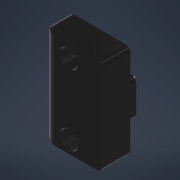
# Autodesk Inventor part: USBCClamp
Saved by Autodesk Inventor 2022 (Build 260153000, 153)
## iProperties
Created: 2021-10-03
Part Number: USBCClamp
Material: Generic
Document SubType Name: Modeling
Designer: trl121
Density: 1 g/cm^3
Appearance: Default
Author: trl121
Autodesk Inventor part; units mm, degrees
ref_plane "YZ Plane" through (0, 0, 0) normal (1, 0, 0) x (0, 1, 0)
ref_plane "XZ Plane" through (0, 0, 0) normal (0, 1, 0) x (-1, 0, 0)
ref_plane "Work Plane1" through (-169.39, -1.905, -0.5195) normal (-1, 0, 0) x (0, -1, 0)
sketch "Sketch1" plane through (-169.39, -1.905, -0.5195) normal (-1, 0, 0) x (0, -1, 0)
  arc A0 (80.1963, 0.7214) -> (80.1963, 3.3714) centre (80.1963, 2.0464) ccw construction
  line L0 (80.1963, 0.7214) -> (74.5063, 0.7214) construction
  arc A1 (74.5063, 3.3714) -> (74.5063, 0.7214) centre (74.5063, 2.0464) ccw construction
  line L1 (74.5063, 3.3714) -> (80.1963, 3.3714) construction
  line L2 (83.7013, -1.7636) -> (71.0013, -1.7636) construction
  arc A2 (83.7013, -1.7636) -> (84.9713, -0.4936) centre (83.7013, -0.4936) ccw construction
  line L3 (84.9713, 5.8564) -> (84.9713, -0.4936) construction
  line L4 (69.7313, -0.4936) -> (69.7313, 5.8564) construction
  arc A3 (69.7313, -0.4936) -> (71.0013, -1.7636) centre (71.0013, -0.4936) ccw construction
  line L5 (69.7313, 5.8564) -> (60.8413, 5.8564) construction
  line L6 (60.8413, 5.8564) -> (60.8413, 12.4375) construction
  line L7 (60.8413, 17.5175) -> (60.8413, 12.4375) construction
  line L8 (93.8613, 5.8564) -> (84.9713, 5.8564) construction
  line L9 (93.8613, 12.4375) -> (93.8613, 5.8564) construction
  line L10 (93.8613, 12.4375) -> (93.8613, 17.5175) construction
  line L11 (93.6613, 17.5175) -> (93.6613, 7.8564)
  line L12 (93.6613, 7.8564) -> (83.7013, 7.8564)
  line L13 (61.0413, 17.5175) -> (61.0413, 7.8564)
  line L14 (61.0413, 7.8564) -> (71.0013, 7.8564)
  line L15 (61.0413, 17.5175) -> (93.6613, 17.5175)
  line L16 (80.1963, 2.0464) -> (74.5063, 2.0464) construction
  line L17 (83.7013, 5.8564) -> (71.0013, 5.8564)
  line L18 (83.7013, 7.8564) -> (83.7013, 5.8564)
  line L19 (71.0013, 5.8564) -> (71.0013, 7.8564)
  point P0 (-1.905, 0.5195)
  dimension "d0" = 2
  dimension "d1" = 0.2
  dimension "d2" = 0.2
  dimension "d3" = 1.27
  dimension "d4" = 1.27
  constraints: 18 end point, 3 perpendicular, 3 vertical, 2 horizontal, 2 horizontal alignment, 2 vertical alignment, 1 collinear, 1 parallel, 1 other
  measures "d0" distance between parallel lines of L8 L12
  measures "d1" distance between parallel lines of L9 L11
  measures "d2" distance between parallel lines of L6 L13
  measures "d3" distance between parallel lines of L18 L3
  measures "d4" distance between parallel lines of L19 L4
extrude "Body" add sketch "Sketch1" against normal blind 20.955
sketch "Sketch2" plane through (-169.39, -95.5663, 16.998) normal (0, 0, 1) x (1, 0, 0)
  circle A0 centre (9.525, 4.245) radius 1.6 projected
  circle A1 centre (9.525, 28.375) radius 1.6 projected
  point P0 (169.39, 95.5663)
extrude "ScrewHoles" cut sketch "Sketch2" against normal through all
sketch "Sketch3" plane through (-169.39, -95.5663, 16.998) normal (0, 0, 1) x (1, 0, 0)
  circle A0 centre (9.525, 4.245) radius 1.6 construction
  circle A1 centre (9.525, 4.245) radius 3.175
  circle A2 centre (9.525, 28.375) radius 3.175
  circle A3 centre (9.525, 28.375) radius 1.6 construction
  point P0 (169.39, 95.5663)
  dimension "d9" = 6.35
  constraints: 2 centre point, 1 coincident, 1 concentric, 1 equal radius
  measures "d9" diameter of A1
extrude "ScrewHeadCut" cut sketch "Sketch3" against normal blind 4.445
sketch "Sketch4" plane through (-169.39, -85.6063, 5.3369) normal (0, 0, -1) x (-1, 0, 0)
  line L0 (0, 12.7) -> (0, 0) construction
  line L1 (0, 12.7) -> (-20.955, 12.7) construction
  line L2 (-20.955, 0) -> (-20.955, 12.7) construction
  line L3 (0, 0) -> (-20.955, 0) construction
  line L4 (-0.6985, 12.319) -> (-1.9685, 12.319)
  line L5 (-1.9685, 12.319) -> (-1.9685, 11.049)
  line L6 (-1.9685, 11.049) -> (-0.6985, 11.049)
  line L7 (-0.6985, 11.049) -> (-0.6985, 12.319)
  line L8 (-2.2225, 12.319) -> (-3.4925, 12.319)
  line L9 (-3.4925, 12.319) -> (-3.4925, 11.049)
  line L10 (-3.4925, 11.049) -> (-2.2225, 11.049)
  line L11 (-2.2225, 11.049) -> (-2.2225, 12.319)
  line L12 (-3.7465, 12.319) -> (-5.0165, 12.319)
  line L13 (-5.0165, 12.319) -> (-5.0165, 11.049)
  line L14 (-5.0165, 11.049) -> (-3.7465, 11.049)
  line L15 (-3.7465, 11.049) -> (-3.7465, 12.319)
  line L16 (-5.2705, 12.319) -> (-6.5405, 12.319)
  line L17 (-6.5405, 12.319) -> (-6.5405, 11.049)
  line L18 (-6.5405, 11.049) -> (-5.2705, 11.049)
  line L19 (-5.2705, 11.049) -> (-5.2705, 12.319)
  line L20 (-6.7945, 12.319) -> (-8.0645, 12.319)
  line L21 (-8.0645, 12.319) -> (-8.0645, 11.049)
  line L22 (-8.0645, 11.049) -> (-6.7945, 11.049)
  line L23 (-6.7945, 11.049) -> (-6.7945, 12.319)
  line L24 (-8.3185, 12.319) -> (-9.5885, 12.319)
  line L25 (-9.5885, 12.319) -> (-9.5885, 11.049)
  line L26 (-9.5885, 11.049) -> (-8.3185, 11.049)
  line L27 (-8.3185, 11.049) -> (-8.3185, 12.319)
  line L28 (-9.8425, 12.319) -> (-11.1125, 12.319)
  line L29 (-11.1125, 12.319) -> (-11.1125, 11.049)
  line L30 (-11.1125, 11.049) -> (-9.8425, 11.049)
  line L31 (-9.8425, 11.049) -> (-9.8425, 12.319)
  line L32 (-11.3665, 12.319) -> (-12.6365, 12.319)
  line L33 (-12.6365, 12.319) -> (-12.6365, 11.049)
  line L34 (-12.6365, 11.049) -> (-11.3665, 11.049)
  line L35 (-11.3665, 11.049) -> (-11.3665, 12.319)
  line L36 (-12.8905, 12.319) -> (-14.1605, 12.319)
  line L37 (-14.1605, 12.319) -> (-14.1605, 11.049)
  line L38 (-14.1605, 11.049) -> (-12.8905, 11.049)
  line L39 (-12.8905, 11.049) -> (-12.8905, 12.319)
  line L40 (-14.4145, 12.319) -> (-15.6845, 12.319)
  line L41 (-15.6845, 12.319) -> (-15.6845, 11.049)
  line L42 (-15.6845, 11.049) -> (-14.4145, 11.049)
  line L43 (-14.4145, 11.049) -> (-14.4145, 12.319)
  line L44 (-15.9385, 12.319) -> (-17.2085, 12.319)
  line L45 (-17.2085, 12.319) -> (-17.2085, 11.049)
  line L46 (-17.2085, 11.049) -> (-15.9385, 11.049)
  line L47 (-15.9385, 11.049) -> (-15.9385, 12.319)
  line L48 (-0.6985, 10.795) -> (-1.9685, 10.795)
  line L49 (-1.9685, 10.795) -> (-1.9685, 9.525)
  line L50 (-1.9685, 9.525) -> (-0.6985, 9.525)
  line L51 (-0.6985, 9.525) -> (-0.6985, 10.795)
  line L52 (-2.2225, 10.795) -> (-3.4925, 10.795)
  line L53 (-3.4925, 10.795) -> (-3.4925, 9.525)
  line L54 (-3.4925, 9.525) -> (-2.2225, 9.525)
  line L55 (-2.2225, 9.525) -> (-2.2225, 10.795)
  line L56 (-3.7465, 10.795) -> (-5.0165, 10.795)
  line L57 (-5.0165, 10.795) -> (-5.0165, 9.525)
  line L58 (-5.0165, 9.525) -> (-3.7465, 9.525)
  line L59 (-3.7465, 9.525) -> (-3.7465, 10.795)
  line L60 (-5.2705, 10.795) -> (-6.5405, 10.795)
  line L61 (-6.5405, 10.795) -> (-6.5405, 9.525)
  line L62 (-6.5405, 9.525) -> (-5.2705, 9.525)
  line L63 (-5.2705, 9.525) -> (-5.2705, 10.795)
  line L64 (-6.7945, 10.795) -> (-8.0645, 10.795)
  line L65 (-8.0645, 10.795) -> (-8.0645, 9.525)
  line L66 (-8.0645, 9.525) -> (-6.7945, 9.525)
  line L67 (-6.7945, 9.525) -> (-6.7945, 10.795)
  line L68 (-8.3185, 10.795) -> (-9.5885, 10.795)
  line L69 (-9.5885, 10.795) -> (-9.5885, 9.525)
  line L70 (-9.5885, 9.525) -> (-8.3185, 9.525)
  line L71 (-8.3185, 9.525) -> (-8.3185, 10.795)
  line L72 (-9.8425, 10.795) -> (-11.1125, 10.795)
  line L73 (-11.1125, 10.795) -> (-11.1125, 9.525)
  line L74 (-11.1125, 9.525) -> (-9.8425, 9.525)
  line L75 (-9.8425, 9.525) -> (-9.8425, 10.795)
  line L76 (-11.3665, 10.795) -> (-12.6365, 10.795)
  line L77 (-12.6365, 10.795) -> (-12.6365, 9.525)
  line L78 (-12.6365, 9.525) -> (-11.3665, 9.525)
  line L79 (-11.3665, 9.525) -> (-11.3665, 10.795)
  line L80 (-12.8905, 10.795) -> (-14.1605, 10.795)
  line L81 (-14.1605, 10.795) -> (-14.1605, 9.525)
  line L82 (-14.1605, 9.525) -> (-12.8905, 9.525)
  line L83 (-12.8905, 9.525) -> (-12.8905, 10.795)
  line L84 (-14.4145, 10.795) -> (-15.6845, 10.795)
  line L85 (-15.6845, 10.795) -> (-15.6845, 9.525)
  line L86 (-15.6845, 9.525) -> (-14.4145, 9.525)
  line L87 (-14.4145, 9.525) -> (-14.4145, 10.795)
  line L88 (-15.9385, 10.795) -> (-17.2085, 10.795)
  line L89 (-17.2085, 10.795) -> (-17.2085, 9.525)
  line L90 (-17.2085, 9.525) -> (-15.9385, 9.525)
  line L91 (-15.9385, 9.525) -> (-15.9385, 10.795)
  line L92 (-0.6985, 9.271) -> (-1.9685, 9.271)
  line L93 (-1.9685, 9.271) -> (-1.9685, 8.001)
  line L94 (-1.9685, 8.001) -> (-0.6985, 8.001)
  line L95 (-0.6985, 8.001) -> (-0.6985, 9.271)
  line L96 (-2.2225, 9.271) -> (-3.4925, 9.271)
  line L97 (-3.4925, 9.271) -> (-3.4925, 8.001)
  line L98 (-3.4925, 8.001) -> (-2.2225, 8.001)
  line L99 (-2.2225, 8.001) -> (-2.2225, 9.271)
  line L100 (-3.7465, 9.271) -> (-5.0165, 9.271)
  line L101 (-5.0165, 9.271) -> (-5.0165, 8.001)
  line L102 (-5.0165, 8.001) -> (-3.7465, 8.001)
  line L103 (-3.7465, 8.001) -> (-3.7465, 9.271)
  line L104 (-5.2705, 9.271) -> (-6.5405, 9.271)
  line L105 (-6.5405, 9.271) -> (-6.5405, 8.001)
  line L106 (-6.5405, 8.001) -> (-5.2705, 8.001)
  line L107 (-5.2705, 8.001) -> (-5.2705, 9.271)
  line L108 (-6.7945, 9.271) -> (-8.0645, 9.271)
  line L109 (-8.0645, 9.271) -> (-8.0645, 8.001)
  line L110 (-8.0645, 8.001) -> (-6.7945, 8.001)
  line L111 (-6.7945, 8.001) -> (-6.7945, 9.271)
  line L112 (-8.3185, 9.271) -> (-9.5885, 9.271)
  line L113 (-9.5885, 9.271) -> (-9.5885, 8.001)
  line L114 (-9.5885, 8.001) -> (-8.3185, 8.001)
  line L115 (-8.3185, 8.001) -> (-8.3185, 9.271)
  line L116 (-9.8425, 9.271) -> (-11.1125, 9.271)
  line L117 (-11.1125, 9.271) -> (-11.1125, 8.001)
  line L118 (-11.1125, 8.001) -> (-9.8425, 8.001)
  line L119 (-9.8425, 8.001) -> (-9.8425, 9.271)
  line L120 (-11.3665, 9.271) -> (-12.6365, 9.271)
  line L121 (-12.6365, 9.271) -> (-12.6365, 8.001)
  line L122 (-12.6365, 8.001) -> (-11.3665, 8.001)
  line L123 (-11.3665, 8.001) -> (-11.3665, 9.271)
  line L124 (-12.8905, 9.271) -> (-14.1605, 9.271)
  line L125 (-14.1605, 9.271) -> (-14.1605, 8.001)
  line L126 (-14.1605, 8.001) -> (-12.8905, 8.001)
  line L127 (-12.8905, 8.001) -> (-12.8905, 9.271)
  line L128 (-14.4145, 9.271) -> (-15.6845, 9.271)
  line L129 (-15.6845, 9.271) -> (-15.6845, 8.001)
  line L130 (-15.6845, 8.001) -> (-14.4145, 8.001)
  line L131 (-14.4145, 8.001) -> (-14.4145, 9.271)
  line L132 (-15.9385, 9.271) -> (-17.2085, 9.271)
  line L133 (-17.2085, 9.271) -> (-17.2085, 8.001)
  line L134 (-17.2085, 8.001) -> (-15.9385, 8.001)
  line L135 (-15.9385, 8.001) -> (-15.9385, 9.271)
  line L136 (-0.6985, 7.747) -> (-1.9685, 7.747)
  line L137 (-1.9685, 7.747) -> (-1.9685, 6.477)
  line L138 (-1.9685, 6.477) -> (-0.6985, 6.477)
  line L139 (-0.6985, 6.477) -> (-0.6985, 7.747)
  line L140 (-2.2225, 7.747) -> (-3.4925, 7.747)
  line L141 (-3.4925, 7.747) -> (-3.4925, 6.477)
  line L142 (-3.4925, 6.477) -> (-2.2225, 6.477)
  line L143 (-2.2225, 6.477) -> (-2.2225, 7.747)
  line L144 (-3.7465, 7.747) -> (-5.0165, 7.747)
  line L145 (-5.0165, 7.747) -> (-5.0165, 6.477)
  line L146 (-5.0165, 6.477) -> (-3.7465, 6.477)
  line L147 (-3.7465, 6.477) -> (-3.7465, 7.747)
  line L148 (-5.2705, 7.747) -> (-6.5405, 7.747)
  line L149 (-6.5405, 7.747) -> (-6.5405, 6.477)
  line L150 (-6.5405, 6.477) -> (-5.2705, 6.477)
  line L151 (-5.2705, 6.477) -> (-5.2705, 7.747)
  line L152 (-6.7945, 7.747) -> (-8.0645, 7.747)
  line L153 (-8.0645, 7.747) -> (-8.0645, 6.477)
  line L154 (-8.0645, 6.477) -> (-6.7945, 6.477)
  line L155 (-6.7945, 6.477) -> (-6.7945, 7.747)
  line L156 (-8.3185, 7.747) -> (-9.5885, 7.747)
  line L157 (-9.5885, 7.747) -> (-9.5885, 6.477)
  line L158 (-9.5885, 6.477) -> (-8.3185, 6.477)
  line L159 (-8.3185, 6.477) -> (-8.3185, 7.747)
  line L160 (-9.8425, 7.747) -> (-11.1125, 7.747)
  line L161 (-11.1125, 7.747) -> (-11.1125, 6.477)
  line L162 (-11.1125, 6.477) -> (-9.8425, 6.477)
  line L163 (-9.8425, 6.477) -> (-9.8425, 7.747)
  line L164 (-11.3665, 7.747) -> (-12.6365, 7.747)
  line L165 (-12.6365, 7.747) -> (-12.6365, 6.477)
  line L166 (-12.6365, 6.477) -> (-11.3665, 6.477)
  line L167 (-11.3665, 6.477) -> (-11.3665, 7.747)
  line L168 (-12.8905, 7.747) -> (-14.1605, 7.747)
  line L169 (-14.1605, 7.747) -> (-14.1605, 6.477)
  line L170 (-14.1605, 6.477) -> (-12.8905, 6.477)
  line L171 (-12.8905, 6.477) -> (-12.8905, 7.747)
  line L172 (-14.4145, 7.747) -> (-15.6845, 7.747)
  line L173 (-15.6845, 7.747) -> (-15.6845, 6.477)
  line L174 (-15.6845, 6.477) -> (-14.4145, 6.477)
  line L175 (-14.4145, 6.477) -> (-14.4145, 7.747)
  line L176 (-15.9385, 7.747) -> (-17.2085, 7.747)
  line L177 (-17.2085, 7.747) -> (-17.2085, 6.477)
  line L178 (-17.2085, 6.477) -> (-15.9385, 6.477)
  line L179 (-15.9385, 6.477) -> (-15.9385, 7.747)
  line L180 (-0.6985, 6.223) -> (-1.9685, 6.223)
  line L181 (-1.9685, 6.223) -> (-1.9685, 4.953)
  line L182 (-1.9685, 4.953) -> (-0.6985, 4.953)
  line L183 (-0.6985, 4.953) -> (-0.6985, 6.223)
  line L184 (-2.2225, 6.223) -> (-3.4925, 6.223)
  line L185 (-3.4925, 6.223) -> (-3.4925, 4.953)
  line L186 (-3.4925, 4.953) -> (-2.2225, 4.953)
  line L187 (-2.2225, 4.953) -> (-2.2225, 6.223)
  line L188 (-3.7465, 6.223) -> (-5.0165, 6.223)
  line L189 (-5.0165, 6.223) -> (-5.0165, 4.953)
  line L190 (-5.0165, 4.953) -> (-3.7465, 4.953)
  line L191 (-3.7465, 4.953) -> (-3.7465, 6.223)
  line L192 (-5.2705, 6.223) -> (-6.5405, 6.223)
  line L193 (-6.5405, 6.223) -> (-6.5405, 4.953)
  line L194 (-6.5405, 4.953) -> (-5.2705, 4.953)
  line L195 (-5.2705, 4.953) -> (-5.2705, 6.223)
  line L196 (-6.7945, 6.223) -> (-8.0645, 6.223)
  line L197 (-8.0645, 6.223) -> (-8.0645, 4.953)
  line L198 (-8.0645, 4.953) -> (-6.7945, 4.953)
  line L199 (-6.7945, 4.953) -> (-6.7945, 6.223)
  line L200 (-8.3185, 6.223) -> (-9.5885, 6.223)
  line L201 (-9.5885, 6.223) -> (-9.5885, 4.953)
  line L202 (-9.5885, 4.953) -> (-8.3185, 4.953)
  line L203 (-8.3185, 4.953) -> (-8.3185, 6.223)
  line L204 (-9.8425, 6.223) -> (-11.1125, 6.223)
  line L205 (-11.1125, 6.223) -> (-11.1125, 4.953)
  line L206 (-11.1125, 4.953) -> (-9.8425, 4.953)
  line L207 (-9.8425, 4.953) -> (-9.8425, 6.223)
  line L208 (-11.3665, 6.223) -> (-12.6365, 6.223)
  line L209 (-12.6365, 6.223) -> (-12.6365, 4.953)
  line L210 (-12.6365, 4.953) -> (-11.3665, 4.953)
  line L211 (-11.3665, 4.953) -> (-11.3665, 6.223)
  line L212 (-12.8905, 6.223) -> (-14.1605, 6.223)
  line L213 (-14.1605, 6.223) -> (-14.1605, 4.953)
  line L214 (-14.1605, 4.953) -> (-12.8905, 4.953)
  line L215 (-12.8905, 4.953) -> (-12.8905, 6.223)
  line L216 (-14.4145, 6.223) -> (-15.6845, 6.223)
  line L217 (-15.6845, 6.223) -> (-15.6845, 4.953)
  line L218 (-15.6845, 4.953) -> (-14.4145, 4.953)
  line L219 (-14.4145, 4.953) -> (-14.4145, 6.223)
  line L220 (-15.9385, 6.223) -> (-17.2085, 6.223)
  line L221 (-17.2085, 6.223) -> (-17.2085, 4.953)
  line L222 (-17.2085, 4.953) -> (-15.9385, 4.953)
  line L223 (-15.9385, 4.953) -> (-15.9385, 6.223)
  line L224 (-0.6985, 4.699) -> (-1.9685, 4.699)
  line L225 (-1.9685, 4.699) -> (-1.9685, 3.429)
  line L226 (-1.9685, 3.429) -> (-0.6985, 3.429)
  line L227 (-0.6985, 3.429) -> (-0.6985, 4.699)
  line L228 (-2.2225, 4.699) -> (-3.4925, 4.699)
  line L229 (-3.4925, 4.699) -> (-3.4925, 3.429)
  line L230 (-3.4925, 3.429) -> (-2.2225, 3.429)
  line L231 (-2.2225, 3.429) -> (-2.2225, 4.699)
  line L232 (-3.7465, 4.699) -> (-5.0165, 4.699)
  line L233 (-5.0165, 4.699) -> (-5.0165, 3.429)
  line L234 (-5.0165, 3.429) -> (-3.7465, 3.429)
  line L235 (-3.7465, 3.429) -> (-3.7465, 4.699)
  line L236 (-5.2705, 4.699) -> (-6.5405, 4.699)
  line L237 (-6.5405, 4.699) -> (-6.5405, 3.429)
  line L238 (-6.5405, 3.429) -> (-5.2705, 3.429)
  line L239 (-5.2705, 3.429) -> (-5.2705, 4.699)
  line L240 (-6.7945, 4.699) -> (-8.0645, 4.699)
  line L241 (-8.0645, 4.699) -> (-8.0645, 3.429)
  line L242 (-8.0645, 3.429) -> (-6.7945, 3.429)
  line L243 (-6.7945, 3.429) -> (-6.7945, 4.699)
  line L244 (-8.3185, 4.699) -> (-9.5885, 4.699)
  line L245 (-9.5885, 4.699) -> (-9.5885, 3.429)
  line L246 (-9.5885, 3.429) -> (-8.3185, 3.429)
  line L247 (-8.3185, 3.429) -> (-8.3185, 4.699)
  line L248 (-9.8425, 4.699) -> (-11.1125, 4.699)
  line L249 (-11.1125, 4.699) -> (-11.1125, 3.429)
  line L250 (-11.1125, 3.429) -> (-9.8425, 3.429)
  line L251 (-9.8425, 3.429) -> (-9.8425, 4.699)
  line L252 (-11.3665, 4.699) -> (-12.6365, 4.699)
  line L253 (-12.6365, 4.699) -> (-12.6365, 3.429)
  line L254 (-12.6365, 3.429) -> (-11.3665, 3.429)
  line L255 (-11.3665, 3.429) -> (-11.3665, 4.699)
  line L256 (-12.8905, 4.699) -> (-14.1605, 4.699)
  line L257 (-14.1605, 4.699) -> (-14.1605, 3.429)
  line L258 (-14.1605, 3.429) -> (-12.8905, 3.429)
  line L259 (-12.8905, 3.429) -> (-12.8905, 4.699)
  line L260 (-14.4145, 4.699) -> (-15.6845, 4.699)
  line L261 (-15.6845, 4.699) -> (-15.6845, 3.429)
  line L262 (-15.6845, 3.429) -> (-14.4145, 3.429)
  line L263 (-14.4145, 3.429) -> (-14.4145, 4.699)
  line L264 (-15.9385, 4.699) -> (-17.2085, 4.699)
  line L265 (-17.2085, 4.699) -> (-17.2085, 3.429)
  line L266 (-17.2085, 3.429) -> (-15.9385, 3.429)
  line L267 (-15.9385, 3.429) -> (-15.9385, 4.699)
  line L268 (-0.6985, 3.175) -> (-1.9685, 3.175)
  line L269 (-1.9685, 3.175) -> (-1.9685, 1.905)
  line L270 (-1.9685, 1.905) -> (-0.6985, 1.905)
  line L271 (-0.6985, 1.905) -> (-0.6985, 3.175)
  line L272 (-2.2225, 3.175) -> (-3.4925, 3.175)
  line L273 (-3.4925, 3.175) -> (-3.4925, 1.905)
  line L274 (-3.4925, 1.905) -> (-2.2225, 1.905)
  line L275 (-2.2225, 1.905) -> (-2.2225, 3.175)
  line L276 (-3.7465, 3.175) -> (-5.0165, 3.175)
  line L277 (-5.0165, 3.175) -> (-5.0165, 1.905)
  line L278 (-5.0165, 1.905) -> (-3.7465, 1.905)
  line L279 (-3.7465, 1.905) -> (-3.7465, 3.175)
  line L280 (-5.2705, 3.175) -> (-6.5405, 3.175)
  line L281 (-6.5405, 3.175) -> (-6.5405, 1.905)
  line L282 (-6.5405, 1.905) -> (-5.2705, 1.905)
  line L283 (-5.2705, 1.905) -> (-5.2705, 3.175)
  line L284 (-6.7945, 3.175) -> (-8.0645, 3.175)
  line L285 (-8.0645, 3.175) -> (-8.0645, 1.905)
  line L286 (-8.0645, 1.905) -> (-6.7945, 1.905)
  line L287 (-6.7945, 1.905) -> (-6.7945, 3.175)
  line L288 (-8.3185, 3.175) -> (-9.5885, 3.175)
  line L289 (-9.5885, 3.175) -> (-9.5885, 1.905)
  line L290 (-9.5885, 1.905) -> (-8.3185, 1.905)
  line L291 (-8.3185, 1.905) -> (-8.3185, 3.175)
  line L292 (-9.8425, 3.175) -> (-11.1125, 3.175)
  line L293 (-11.1125, 3.175) -> (-11.1125, 1.905)
  line L294 (-11.1125, 1.905) -> (-9.8425, 1.905)
  line L295 (-9.8425, 1.905) -> (-9.8425, 3.175)
  line L296 (-11.3665, 3.175) -> (-12.6365, 3.175)
  line L297 (-12.6365, 3.175) -> (-12.6365, 1.905)
  line L298 (-12.6365, 1.905) -> (-11.3665, 1.905)
  line L299 (-11.3665, 1.905) -> (-11.3665, 3.175)
  line L300 (-12.8905, 3.175) -> (-14.1605, 3.175)
  line L301 (-14.1605, 3.175) -> (-14.1605, 1.905)
  line L302 (-14.1605, 1.905) -> (-12.8905, 1.905)
  line L303 (-12.8905, 1.905) -> (-12.8905, 3.175)
  line L304 (-14.4145, 3.175) -> (-15.6845, 3.175)
  line L305 (-15.6845, 3.175) -> (-15.6845, 1.905)
  line L306 (-15.6845, 1.905) -> (-14.4145, 1.905)
  line L307 (-14.4145, 1.905) -> (-14.4145, 3.175)
  line L308 (-15.9385, 3.175) -> (-17.2085, 3.175)
  line L309 (-17.2085, 3.175) -> (-17.2085, 1.905)
  line L310 (-17.2085, 1.905) -> (-15.9385, 1.905)
  line L311 (-15.9385, 1.905) -> (-15.9385, 3.175)
  line L312 (0, 0) -> (-20.955, 12.7) construction
  line L313 (-20.955, 0) -> (0, 12.7) construction
  line L314 (-17.4625, 12.319) -> (-18.7325, 12.319)
  line L315 (-18.7325, 12.319) -> (-18.7325, 11.049)
  line L316 (-18.7325, 11.049) -> (-17.4625, 11.049)
  line L317 (-17.4625, 11.049) -> (-17.4625, 12.319)
  line L318 (-17.4625, 10.795) -> (-18.7325, 10.795)
  line L319 (-18.7325, 10.795) -> (-18.7325, 9.525)
  line L320 (-18.7325, 9.525) -> (-17.4625, 9.525)
  line L321 (-17.4625, 9.525) -> (-17.4625, 10.795)
  line L322 (-17.4625, 9.271) -> (-18.7325, 9.271)
  line L323 (-18.7325, 9.271) -> (-18.7325, 8.001)
  line L324 (-18.7325, 8.001) -> (-17.4625, 8.001)
  line L325 (-17.4625, 8.001) -> (-17.4625, 9.271)
  line L326 (-17.4625, 7.747) -> (-18.7325, 7.747)
  line L327 (-18.7325, 7.747) -> (-18.7325, 6.477)
  line L328 (-18.7325, 6.477) -> (-17.4625, 6.477)
  line L329 (-17.4625, 6.477) -> (-17.4625, 7.747)
  line L330 (-17.4625, 6.223) -> (-18.7325, 6.223)
  line L331 (-18.7325, 6.223) -> (-18.7325, 4.953)
  line L332 (-18.7325, 4.953) -> (-17.4625, 4.953)
  line L333 (-17.4625, 4.953) -> (-17.4625, 6.223)
  line L334 (-17.4625, 4.699) -> (-18.7325, 4.699)
  line L335 (-18.7325, 4.699) -> (-18.7325, 3.429)
  line L336 (-18.7325, 3.429) -> (-17.4625, 3.429)
  line L337 (-17.4625, 3.429) -> (-17.4625, 4.699)
  line L338 (-17.4625, 3.175) -> (-18.7325, 3.175)
  line L339 (-18.7325, 3.175) -> (-18.7325, 1.905)
  line L340 (-18.7325, 1.905) -> (-17.4625, 1.905)
  line L341 (-17.4625, 1.905) -> (-17.4625, 3.175)
  line L342 (-0.6985, 1.651) -> (-1.9685, 1.651)
  line L343 (-1.9685, 1.651) -> (-1.9685, 0.381)
  line L344 (-1.9685, 0.381) -> (-0.6985, 0.381)
  line L345 (-0.6985, 0.381) -> (-0.6985, 1.651)
  line L346 (-2.2225, 1.651) -> (-3.4925, 1.651)
  line L347 (-3.4925, 1.651) -> (-3.4925, 0.381)
  line L348 (-3.4925, 0.381) -> (-2.2225, 0.381)
  line L349 (-2.2225, 0.381) -> (-2.2225, 1.651)
  line L350 (-3.7465, 1.651) -> (-5.0165, 1.651)
  line L351 (-5.0165, 1.651) -> (-5.0165, 0.381)
  line L352 (-5.0165, 0.381) -> (-3.7465, 0.381)
  line L353 (-3.7465, 0.381) -> (-3.7465, 1.651)
  line L354 (-5.2705, 1.651) -> (-6.5405, 1.651)
  line L355 (-6.5405, 1.651) -> (-6.5405, 0.381)
  line L356 (-6.5405, 0.381) -> (-5.2705, 0.381)
  line L357 (-5.2705, 0.381) -> (-5.2705, 1.651)
  line L358 (-6.7945, 1.651) -> (-8.0645, 1.651)
  line L359 (-8.0645, 1.651) -> (-8.0645, 0.381)
  line L360 (-8.0645, 0.381) -> (-6.7945, 0.381)
  line L361 (-6.7945, 0.381) -> (-6.7945, 1.651)
  line L362 (-8.3185, 1.651) -> (-9.5885, 1.651)
  line L363 (-9.5885, 1.651) -> (-9.5885, 0.381)
  line L364 (-9.5885, 0.381) -> (-8.3185, 0.381)
  line L365 (-8.3185, 0.381) -> (-8.3185, 1.651)
  line L366 (-9.8425, 1.651) -> (-11.1125, 1.651)
  line L367 (-11.1125, 1.651) -> (-11.1125, 0.381)
  line L368 (-11.1125, 0.381) -> (-9.8425, 0.381)
  line L369 (-9.8425, 0.381) -> (-9.8425, 1.651)
  line L370 (-11.3665, 1.651) -> (-12.6365, 1.651)
  line L371 (-12.6365, 1.651) -> (-12.6365, 0.381)
  line L372 (-12.6365, 0.381) -> (-11.3665, 0.381)
  line L373 (-11.3665, 0.381) -> (-11.3665, 1.651)
  line L374 (-12.8905, 1.651) -> (-14.1605, 1.651)
  line L375 (-14.1605, 1.651) -> (-14.1605, 0.381)
  line L376 (-14.1605, 0.381) -> (-12.8905, 0.381)
  line L377 (-12.8905, 0.381) -> (-12.8905, 1.651)
  line L378 (-14.4145, 1.651) -> (-15.6845, 1.651)
  line L379 (-15.6845, 1.651) -> (-15.6845, 0.381)
  line L380 (-15.6845, 0.381) -> (-14.4145, 0.381)
  line L381 (-14.4145, 0.381) -> (-14.4145, 1.651)
  line L382 (-15.9385, 1.651) -> (-17.2085, 1.651)
  line L383 (-17.2085, 1.651) -> (-17.2085, 0.381)
  line L384 (-17.2085, 0.381) -> (-15.9385, 0.381)
  line L385 (-15.9385, 0.381) -> (-15.9385, 1.651)
  line L386 (-17.4625, 1.651) -> (-18.7325, 1.651)
  line L387 (-18.7325, 1.651) -> (-18.7325, 0.381)
  line L388 (-18.7325, 0.381) -> (-17.4625, 0.381)
  line L389 (-17.4625, 0.381) -> (-17.4625, 1.651)
  line L390 (-18.9865, 12.319) -> (-20.2565, 12.319)
  line L391 (-20.2565, 12.319) -> (-20.2565, 11.049)
  line L392 (-20.2565, 11.049) -> (-18.9865, 11.049)
  line L393 (-18.9865, 11.049) -> (-18.9865, 12.319)
  line L394 (-18.9865, 10.795) -> (-20.2565, 10.795)
  line L395 (-20.2565, 10.795) -> (-20.2565, 9.525)
  line L396 (-20.2565, 9.525) -> (-18.9865, 9.525)
  line L397 (-18.9865, 9.525) -> (-18.9865, 10.795)
  line L398 (-18.9865, 9.271) -> (-20.2565, 9.271)
  line L399 (-20.2565, 9.271) -> (-20.2565, 8.001)
  line L400 (-20.2565, 8.001) -> (-18.9865, 8.001)
  line L401 (-18.9865, 8.001) -> (-18.9865, 9.271)
  line L402 (-18.9865, 7.747) -> (-20.2565, 7.747)
  line L403 (-20.2565, 7.747) -> (-20.2565, 6.477)
  line L404 (-20.2565, 6.477) -> (-18.9865, 6.477)
  line L405 (-18.9865, 6.477) -> (-18.9865, 7.747)
  line L406 (-18.9865, 6.223) -> (-20.2565, 6.223)
  line L407 (-20.2565, 6.223) -> (-20.2565, 4.953)
  line L408 (-20.2565, 4.953) -> (-18.9865, 4.953)
  line L409 (-18.9865, 4.953) -> (-18.9865, 6.223)
  line L410 (-18.9865, 4.699) -> (-20.2565, 4.699)
  line L411 (-20.2565, 4.699) -> (-20.2565, 3.429)
  line L412 (-20.2565, 3.429) -> (-18.9865, 3.429)
  line L413 (-18.9865, 3.429) -> (-18.9865, 4.699)
  line L414 (-18.9865, 3.175) -> (-20.2565, 3.175)
  line L415 (-20.2565, 3.175) -> (-20.2565, 1.905)
  line L416 (-20.2565, 1.905) -> (-18.9865, 1.905)
  line L417 (-18.9865, 1.905) -> (-18.9865, 3.175)
  line L418 (-18.9865, 1.651) -> (-20.2565, 1.651)
  line L419 (-20.2565, 1.651) -> (-20.2565, 0.381)
  line L420 (-20.2565, 0.381) -> (-18.9865, 0.381)
  line L421 (-18.9865, 0.381) -> (-18.9865, 1.651)
  line L422 (-10.4775, 6.223) -> (-10.4775, 6.477) construction
  point P0 (-169.39, 85.6063)
  point P1 (-10.4775, 6.35)
  point P2 (-10.4775, 6.35)
  dimension "d12" = 1.27
  dimension "d15" = 1.524
  dimension "d18" = 1.524
  constraints: 838 end point, 5 midpoint, 2 collinear, 2 horizontal, 2 parallel, 2 perpendicular, 1 vertical, 822 other
  measures "d12" distance of L5.end L6.end
  measures "d15" distance of L4.start L8.start
  measures "d18" distance of L4.start L48.start
extrude "BottomStuds" add sketch "Sketch4" along normal blind 50.8 draft -35
fillet "Fillets" radius 5.08 1 edges at (-169.39, -79.2563, 16.998)
fillet "Fillets" radius 1.905 8 edges at (-169.39, -95.5663, 12.1675) (-169.39, -62.9463, 12.1675) (-148.435, -95.5663, 12.1675) (-148.435, -62.9463, 12.1675) (-169.39, -85.6063, 6.3369) (-169.39, -72.9063, 6.3369) (-148.435, -85.6063, 6.3369) (-148.435, -72.9063, 6.3369)
equation "\"d4\" = d3"
body "Solid1"
